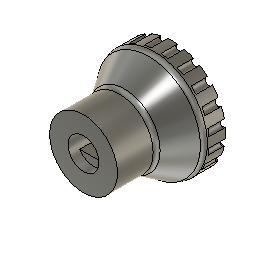
MIWPS Button v9 (Autodesk Fusion 360 design; units mm, degrees)
Autodesk Fusion 360 part; units mm, degrees
sketch "button" plane through (0, 0, 0) normal (0, 0, 1) x (1, 0, 0)
  line L0 (0, 0) -> (7, 0)
  line L1 (7, 0) -> (7, 8)
  line L2 (7, 8) -> (11, 14)
  line L3 (11, 14) -> (11, 18)
  line L4 (11, 18) -> (7, 18)
  line L5 (7, 18) -> (0, 16)
  line L6 (0, 0) -> (3.2, 0)
  line L7 (3.2, 0) -> (3.2, 15)
  line L8 (3.2, 15) -> (0, 15)
  line L9 (0, 15) -> (0, 0)
  line L10 (0, 15) -> (0, 16)
  line L11 (0, 15) -> (3.2, 13.1525)
  line L12 (0, 15) -> (4.1383, 15) construction
  point P0 (7, 8)
  point P1 (7, 18)
  dimension "d6" = 7
  dimension "d7" = 8
  dimension "d10" = 11
  dimension "d12" = 4
  dimension "d14" = 4
  dimension "d15" = 16
  dimension "d16" = 7
  dimension "d17" = 3.2
  dimension "d18" = 15
  dimension "d24" = 30
  dimension "d29" = 6
  constraint coincident L0.start L6.start
  constraint horizontal L0
  constraint perpendicular L0 L1
  constraint coincident P0 L1.end
  constraint vertical L3
  constraint coincident P1 L4.end
  constraint horizontal L6
  constraint vertical L7
  constraint horizontal L8
  constraint vertical L9
  constraint horizontal L12
  constraint coincident L7 L11.end
  constraint perpendicular L3 L4
  measures "d6" distance of L0.start L0.end
  measures "d7" distance of L0.end P0
  measures "d10" horizontal distance of L0.start L2.end
  measures "d12" distance of L3 P1
  measures "d14" distance of L2.end L3.end
  measures "d15" distance of L0.start L5.end
  measures "d16" horizontal distance of P1 L5.end
  measures "d17" distance of L0.start L6.end
  measures "d18" distance of L0.start L8.end
  measures "d24" angle of L11 L12
  measures "d29" vertical distance of P0 L2.end
revolve "Revolve1" add sketch "button" angle 360 about axis through (0, 15, 0) along (0, -1, 0) contours L0 L1 L2 L3 L4 L5 L7 L8 L10 | L7 L8 L11
ref_plane "WorkPlane1" through (0, 2, 0) normal (0, -1, 0) x (0, 0, -1)
sketch "tab" plane through (0, 2, 0) normal (0, -1, 0) x (1, 0, 0)
  line L0 (3.5, -5.6) -> (-3.5, -5.6)
  line L1 (-3.5, -5.6) -> (-3.5, -1.6)
  line L2 (-3.5, -1.6) -> (3.5, -1.6)
  line L3 (3.5, -1.6) -> (3.5, -5.6)
  line L4 (3.5, -5.6) -> (-3.5, -1.6) construction
  line L5 (-3.5, -5.6) -> (3.5, -1.6) construction
  circle A0 centre (0, 0) radius 7
  point P0 (0, -3.6)
  dimension "d21" = 7
  dimension "d22" = 4
  dimension "d23" = 3.6
  constraint horizontal L0
  constraint perpendicular L0 L1
  constraint parallel L0 L2
  constraint parallel L1 L3
  constraint coincident L4 P0
  constraint coincident L5 P0
  measures "d21" distance of L1.end L2.end
  measures "d22" distance of L0.end L1.end
  measures "d23" distance of P0 A0.centre
sketch "finger grips" plane through (0, 18, 0) normal (0, 1, 0) x (-1, 0, 0)
  circle A0 centre (0, 0) radius 7
  circle A1 centre (0, 0) radius 11
  line L0 (0.0163, 7) -> (-1.0034, 10.9541)
  line L1 (0.9966, 10.9548) -> (0.0163, 7)
  arc A2 (0.9966, 10.9548) -> (2.3995, 10.7351) centre (1.7358, 11.0855) ccw
  dimension "d37" = 2
  dimension "d39" = 1.42
  constraint coincident A0 L0.start
  constraint coincident A1 L0.end
  constraint coincident A1 L1.start
  constraint coincident A1 A2.end
  measures "d37" distance of L0.end L1.start
  measures "d39" distance of L1.start A2.end
extrude "Extrude1" add sketch "finger grips" along normal blind 0.4 contours A1 L0 L1
pattern_circular "C-Pattern1" count 20 over 360 about axis through (0, 1.75, 0) along (0, 1, 0) of "Extrude1"
extrude "Extrude2" add sketch "tab" against normal blind 12 contours L0 L1 L2 L3
fillet "Fillet1" radius 2 1 edges at (-10.2556, 14, -3.9778)
fillet "Fillet2" radius 2 1 edges at (-6.5263, 8, -2.5313)
extrude "Extrude3" cut sketch "finger grips" against normal blind 3 contours A1 A2
pattern_circular "C-Pattern2" count 20 over 360 about axis through (0, 1.75, 0) along (0, 1, 0) of "Extrude3"
named bodies: "MIWPS Button"
